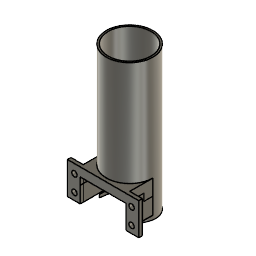
Ball storage (Pei yu design) (Autodesk Fusion 360 design; units mm, degrees)
part number: 2026-01-22-19-12-14-091
part number: 2026-01-22-19-45-21-594
part number: 2026-01-22-20-39-39-913
Autodesk Fusion 360 part; units mm, degrees
note: some values were not read from the file. Set by a fixed rule: which sketch regions a step uses.
sketch "Sketch2" plane through (0, 0, 0) normal (0, 0, 1) x (1, 0, 0)
  circle A0 centre (0, 0) radius 13
  dimension "d2" = 26
  constraint coincident A0.centre origin
  measures "d2" diameter of A0
extrude "Extrude1" add sketch "Sketch2" along normal blind 90 makes body 1
hole "Hole1" at (0, 0, 90) direction (0, 0, -1) diameter 24 depth 90 tip angle 118 bodies 1
sketch "Sketch3" plane through (0, 0, 0) normal (0, 1, 0) x (1, 0, 0)
  line L0 (0, 0) -> (35, 0)
  line L1 (35, 0) -> (35, 15)
  line L2 (35, 15) -> (0, 15)
  line L3 (0, 15) -> (0, 0)
  dimension "d8" = 15
  dimension "d9" = 35
  constraint horizontal L0
  constraint vertical L1
  constraint horizontal L2
  constraint vertical L3
  constraint coincident L0.start L3.end
  measures "d8" distance of L0.start L2.end
  measures "d9" distance of L0.start L0.end
sketch "Sketch5" plane through (0, 0, 0) normal (0, 0, 1) x (1, 0, 0)
  line L0 (15.4956, -21.1773) -> (-24.5044, -21.1773)
  line L1 (-24.5044, -21.1773) -> (-24.5044, -19.1773)
  line L2 (-24.5044, -19.1773) -> (15.4956, -19.1773)
  line L3 (15.4956, -19.1773) -> (15.4956, -21.1773)
  dimension "d14" = 2
  dimension "d15" = 40
  constraint horizontal L0
  constraint vertical L1
  constraint horizontal L2
  constraint vertical L3
  measures "d14" distance of L0.start L2.end
  measures "d15" distance of L0.start L0.end
extrude "Extrude1'" add sketch "Sketch5" along normal blind 18 separate body makes body 2 in component "Component'"
sketch "Sketch6" plane through (0, -14.9073, 0) normal (0, -1, 0) x (1, 0, 0)
  line L0 (-19.946, 13.4469) -> (20.054, 13.4469)
  line L1 (20.054, 13.4469) -> (20.054, 31.4469)
  line L2 (20.054, 31.4469) -> (-19.946, 31.4469)
  line L3 (-19.946, 31.4469) -> (-19.946, 13.4469)
  circle A0 centre (-15.977, 26.4692) radius 1.5
  circle A1 centre (-15.9675, 17.4692) radius 1.5
  line L4 (-21.6195, 22.4566) -> (22.3805, 22.4566)
  line L5 (0.023, 33.6355) -> (0.023, 10)
  line L6 (-15.9839, 33) -> (-15.9609, 11.2428)
  circle A2 centre (16.023, 26.4692) radius 1.5
  circle A3 centre (16.0135, 17.4692) radius 1.5
  dimension "d18" = 3
  dimension "d19" = 3
  dimension "d20" = 9
  dimension "d21" = 16
  constraint perpendicular L1 L4
  constraint perpendicular L0 L5
  constraint coincident A0.centre L6
  constraint coincident A1.centre L6
  constraint symmetric A0 L5 A2
  constraint symmetric A1 L5 A3
  measures "d18" diameter of A0
  measures "d19" diameter of A1
  measures "d20" vertical distance of A0.centre A1.centre
  measures "d21" distance of A0.centre L5
extrude "Extrude2" cut sketch "Sketch6" against normal blind 2 contours A1 L6 | A1 L6 | A0 L6 | A0 L6 | A2 | A3 sketch seen with x (1, 0, 0) y (0, 1, 0) z (0, 0, 1) at (-4.5583, -6.27, -13.4469) bodies 2 in component "Component'"
combine "Combine1" operation add target body 1 tool bodies 2 body 2 seen with x (1, 0, 0) y (0, 1, 0) z (0, 0, 1) at (4.5583, 6.27, 13.4469)
sketch "Sketch7" plane through (0, 0, 31.4469) normal (0, 0, 1) x (-1, 0, 0)
  arc A0 (1.5494, 12.9073) -> (-1.5494, 12.9073) centre (0, 0) ccw
  line L0 (1.5494, 12.9073) -> (19.946, 12.9073)
  line L1 (19.946, 12.9073) -> (19.946, 14.9073)
  line L2 (19.946, 14.9073) -> (-20.054, 14.9073)
  line L3 (-20.054, 14.9073) -> (-20.054, 12.9073)
  line L4 (-20.054, 12.9073) -> (-1.5494, 12.9073)
  line L5 (1.5494, 12.9073) -> (13, 12.9073)
  line L6 (13, 1) -> (9.9168, 8.2831)
  line L7 (9.9168, 8.2831) -> (1.5494, 12.9073)
  line L8 (13, 12.9073) -> (13, 1)
  constraint coincident A0.start L0.start
  constraint coincident L0 L5.end
  constraint perpendicular L5 L8
extrude "Extrude2'" add sketch "Sketch7" against normal blind 18 contours L0 L5 L6 L7 L8 bodies 1
sketch "Sketch9" plane through (0, 0, 0) normal (0, 1, 0) x (1, 0, 0)
sketch "Sketch10" plane through (0, 0, 31.4469) normal (0, 0, 1) x (-1, 0, 0)
  arc A0 (12.9523, 1.1127) -> (-1.5494, 12.9073) centre (0, 0) ccw
  line L0 (12.9523, 1.1127) -> (13, 1)
  line L1 (13, 1) -> (13, 12.9073)
  line L2 (13, 12.9073) -> (19.946, 12.9073)
  line L3 (19.946, 12.9073) -> (19.946, 14.9073)
  line L4 (19.946, 14.9073) -> (-20.054, 14.9073)
  line L5 (-20.054, 14.9073) -> (-20.054, 12.9073)
  line L6 (-20.054, 12.9073) -> (-1.5494, 12.9073)
  line L7 (-1.5494, 12.9073) -> (-13, 12.9073)
  line L8 (-13, 0) -> (-13, 12.9073)
  line L9 (-1.5494, 12.9073) -> (-9, 9)
  line L10 (-9, 9) -> (-13, 0)
  constraint coincident A0.end L6.end
  constraint coincident L6 L7.end
  constraint perpendicular L7 L8
extrude "Extrude3" add sketch "Sketch10" against normal blind 18 contours L6 L7 L8 L9 L10 bodies 1
sketch "Sketch11" plane through (0, 0, 0) normal (1, 0, 0) x (0, 1, 0)
  line L0 (-13, 10) -> (20, -1)
  line L1 (-13, 10) -> (-13, -3)
  line L2 (-13, -3) -> (20, -1)
  constraint vertical L1
extrude "Extrude4" cut sketch "Sketch11" along normal blind 50 draft 1 and the other way blind 18 bodies 1
sketch "Sketch12" plane through (0, 0, 0) normal (1, 0, 0) x (0, 1, 0)
  line L0 (-14, 12) -> (17, 5)
  line L1 (17, 5) -> (18, -4)
  line L2 (18, -4) -> (-15, -4)
  line L3 (-15, -4) -> (-14, 12)
  constraint horizontal L2
extrude "Extrude5" cut sketch "Sketch12" along normal blind 50 and the other way blind 41 bodies 1
sketch "Sketch13" plane through (0, 0, 0) normal (1, 0, 0) x (0, 1, 0)
  line L0 (-14, 13) -> (16, 9)
  line L1 (16, 9) -> (16, -1)
  line L2 (16, -1) -> (-15, -1)
  line L3 (-15, -1) -> (-14, 13)
  constraint vertical L1
  constraint perpendicular L1 L2
extrude "Extrude6" cut sketch "Sketch13" along normal blind 50 and the other way blind 23 bodies 1
sketch "Sketch14" plane through (0, -14.9073, 0) normal (0, -1, 0) x (1, 0, 0)
  circle A0 centre (-15.9675, 17.4692) radius 1.5
  circle A1 centre (16.0135, 17.4692) radius 1.5
  circle A2 centre (-15.977, 26.4692) radius 1.5
  circle A3 centre (16.023, 26.4692) radius 1.5
  line L0 (-19.946, 13.4469) -> (20.054, 13.4469)
  line L1 (20.054, 13.4469) -> (20.054, 31.4469)
  line L2 (20.054, 31.4469) -> (-19.946, 31.4469)
  line L3 (-19.946, 31.4469) -> (-19.946, 13.4469)
  line L4 (-12.7186, 22.5492) -> (12.8697, 22.5492)
  line L5 (12.8697, 22.5492) -> (12.8697, 9.3656)
  line L6 (12.8697, 9.3656) -> (-12.7186, 9.3656)
  line L7 (-12.7186, 9.3656) -> (-12.7186, 22.5492)
  constraint horizontal L4
  constraint vertical L5
  constraint horizontal L6
  constraint vertical L7
extrude "Extrude7" cut sketch "Sketch14" against normal blind 15 contours L0 L4 L5 L7 bodies 1
sketch "Sketch15" plane through (0, 0, 0) normal (0, 0, 1) x (1, 0, 0)
sketch "Sketch16" plane through (0, 0.0927, 0) normal (0, -1, 0) x (1, 0, 0)
  line L0 (-11.9996, 13.4469) -> (-11.9996, 22.5492)
  line L1 (-11.9996, 22.5492) -> (-12.7186, 22.5492)
  line L2 (-12.7186, 22.5492) -> (-12.7186, 13.4469)
  line L3 (-12.7186, 13.4469) -> (-11.9996, 13.4469)
  line L4 (-11.9996, 16.1398) -> (12, 16.1398)
  line L5 (12, 16.1398) -> (12, 10)
  line L6 (12, 10) -> (-11.9996, 10)
  line L7 (-11.9996, 10) -> (-11.9996, 16.1398)
  constraint horizontal L4
  constraint vertical L5
  constraint horizontal L6
  constraint vertical L7
  constraint coincident L0 L4.start
extrude "Extrude8" cut sketch "Sketch16" along normal blind 50 contours L0 L4 L5 L6 L7 bodies 1
sketch "Sketch17" plane through (0, -14.9073, 0) normal (0, -1, 0) x (1, 0, 0)
  line L0 (-12.7186, 13.4469) -> (-12.7186, 22.5492)
  line L1 (-12.7186, 22.5492) -> (12.8697, 22.5492)
  line L2 (12.8697, 22.5492) -> (12.8697, 13.4469)
  line L3 (12.8697, 13.4469) -> (20.054, 13.4469)
  line L4 (20.054, 13.4469) -> (20.054, 31.4469)
  line L5 (20.054, 31.4469) -> (-19.946, 31.4469)
  line L6 (-19.946, 31.4469) -> (-19.946, 13.4469)
  line L7 (-19.946, 13.4469) -> (-12.7186, 13.4469)
  circle A0 centre (16.023, 26.4692) radius 1.5
  circle A1 centre (-15.977, 26.4692) radius 1.5
  circle A2 centre (16.0135, 17.4692) radius 1.5
  circle A3 centre (-15.9675, 17.4692) radius 1.5
  line L8 (-12.7276, 26.5492) -> (12.8697, 26.5492)
  line L9 (12.8697, 26.5492) -> (12.8697, 22.5492)
  line L10 (12.8697, 22.5492) -> (-12.7276, 22.5492)
  line L11 (-12.7276, 22.5492) -> (-12.7276, 26.5492)
  dimension "d44" = 4
  constraint horizontal L8
  constraint vertical L9
  constraint horizontal L10
  constraint vertical L11
  constraint coincident L1.end L2.start
  measures "d44" distance of L8.start L10.end
extrude "Extrude9" cut sketch "Sketch17" against normal blind 10 contours L1 L8 L9 L10 L11 bodies 1
component "Component" placed x (1, 0, 0) y (0, 1, 0) z (0, 0, 1) at (0, 0, 0)
component "Component'" placed x (1, 0, 0) y (0, 1, 0) z (0, 0, 1) at (4.5583, 6.27, 13.4469)
equation "d29 = deg"
